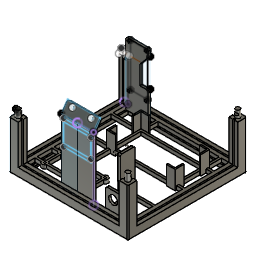
frame_base (Autodesk Fusion 360 design; units mm, degrees)
Autodesk Fusion 360 part; units mm, degrees
note: some values were not read from the file. Chosen so that the rebuilt part matches the saved one: which bodies a step acts on; a direction. Set by a fixed rule: which sketch regions a step uses; the direction of a hole.
sketch "Skizze1" plane through (0, 0, 0) normal (0, 0, 1) x (1, 0, 0)
  line L0 (0, 0) -> (160, 0)
  line L1 (160, 0) -> (160, 160)
  line L2 (160, 160) -> (0, 160)
  line L3 (0, 160) -> (0, 0)
  line L4 (12, 148) -> (148, 148)
  line L5 (148, 148) -> (148, 12)
  line L6 (148, 12) -> (12, 12)
  line L7 (12, 12) -> (12, 148)
  line L8 (12, 148) -> (0, 148)
  line L9 (0, 148) -> (0, 160)
  line L10 (0, 160) -> (12, 160)
  line L11 (12, 160) -> (12, 148)
  line L12 (148, 148) -> (160, 148)
  line L13 (160, 148) -> (160, 160)
  line L14 (160, 160) -> (148, 160)
  line L15 (148, 160) -> (148, 148)
  line L16 (148, 12) -> (160, 12)
  line L17 (160, 12) -> (160, 0)
  line L18 (160, 0) -> (148, 0)
  line L19 (148, 0) -> (148, 12)
  line L20 (12, 12) -> (0, 12)
  line L21 (0, 12) -> (0, 0)
  line L22 (0, 0) -> (12, 0)
  line L23 (12, 0) -> (12, 12)
  circle A0 centre (6, 6) radius 3
  circle A1 centre (154, 6) radius 3
  circle A2 centre (154, 154) radius 3
  circle A3 centre (6, 154) radius 3
  line L24 (154, 148) -> (154, 12) construction
  line L25 (148, 154) -> (12, 154) construction
  line L26 (6, 148) -> (6, 12) construction
  line L27 (12, 6) -> (148, 6) construction
  line L28 (152.9, 150) -> (155.1, 150)
  line L29 (155.1, 150) -> (155.1, 10)
  line L30 (155.1, 10) -> (152.9, 10)
  line L31 (152.9, 10) -> (152.9, 150)
  line L32 (4.9, 150) -> (7.1, 150)
  line L33 (7.1, 150) -> (7.1, 10)
  line L34 (7.1, 10) -> (4.9, 10)
  line L35 (4.9, 10) -> (4.9, 150)
  line L36 (10, 152.9) -> (150, 152.9)
  line L37 (150, 152.9) -> (150, 155.1)
  line L38 (150, 155.1) -> (10, 155.1)
  line L39 (10, 155.1) -> (10, 152.9)
  line L40 (10, 4.9) -> (150, 4.9)
  line L41 (150, 4.9) -> (150, 7.1)
  line L42 (150, 7.1) -> (10, 7.1)
  line L43 (10, 7.1) -> (10, 4.9)
  dimension "d1" = 160
  dimension "d2" = 160
  dimension "d3" = 12
  dimension "d4" = 12
  dimension "d5" = 12
  dimension "d6" = 12
  dimension "d7" = 6
  dimension "d8" = 6
  dimension "d9" = 6
  dimension "d10" = 6
  dimension "d11" = 6
  dimension "d12" = 6
  dimension "d13" = 6
  dimension "d14" = 6
  dimension "d15" = 6
  dimension "d16" = 6
  dimension "d17" = 6
  dimension "d18" = 6
  dimension "d19" = 2.2
  dimension "d20" = 140
  dimension "d21" = 4.9
  dimension "d22" = 10
  dimension "d23" = 2.2
  dimension "d24" = 140
  dimension "d25" = 4.9
  dimension "d26" = 10
  dimension "d27" = 140
  dimension "d28" = 2.2
  dimension "d29" = 10
  dimension "d30" = 4.9
  dimension "d31" = 140
  dimension "d32" = 2.2
  dimension "d33" = 10
  dimension "d34" = 4.9
  constraint horizontal L0
  constraint vertical L1
  constraint horizontal L2
  constraint vertical L3
  constraint coincident L0.start L3.end
  constraint horizontal L4
  constraint vertical L5
  constraint horizontal L6
  constraint vertical L7
  constraint horizontal L8
  constraint vertical L9
  constraint horizontal L10
  constraint vertical L11
  constraint horizontal L12
  constraint vertical L13
  constraint horizontal L14
  constraint vertical L15
  constraint horizontal L16
  constraint vertical L17
  constraint horizontal L18
  constraint vertical L19
  constraint horizontal L20
  constraint vertical L21
  constraint horizontal L22
  constraint vertical L23
  constraint midpoint L12 L24.start
  constraint midpoint L16 L24.end
  constraint midpoint L15 L25.start
  constraint midpoint L11 L25.end
  constraint midpoint L8 L26.start
  constraint midpoint L20 L26.end
  constraint midpoint L23 L27.start
  constraint midpoint L19 L27.end
  constraint horizontal L28
  constraint vertical L29
  constraint horizontal L30
  constraint vertical L31
  constraint horizontal L32
  constraint vertical L33
  constraint horizontal L34
  constraint vertical L35
  constraint horizontal L36
  constraint vertical L37
  constraint horizontal L38
  constraint vertical L39
  constraint horizontal L40
  constraint vertical L41
  constraint horizontal L42
  constraint vertical L43
  measures "d1" distance of L0.start L0.end
  measures "d2" distance of L0.start L2.end
  measures "d3" distance of L3 L7
  measures "d4" distance of L1 L5
  measures "d5" distance of L0 L6
  measures "d6" distance of L2 L4
  measures "d7" diameter of A0
  measures "d8" diameter of A1
  measures "d9" diameter of A2
  measures "d10" diameter of A3
  measures "d11" distance of L3 A0.centre
  measures "d12" distance of L17 A1.centre
  measures "d13" distance of L13 A2.centre
  measures "d14" distance of L3 A3.centre
  measures "d15" distance of L12 A2.centre
  measures "d16" distance of L0 A1.centre
  measures "d17" distance of L22 A0.centre
  measures "d18" distance of L8 A3.centre
  measures "d19" distance of L28.start L28.end
  measures "d20" distance of L28.start L30.end
  measures "d21" distance of L1 L29
  measures "d22" distance of L2 L28
  measures "d23" distance of L32.start L32.end
  measures "d24" distance of L32.start L34.end
  measures "d25" distance of L3 L35
  measures "d26" distance of L2 L32
  measures "d27" distance of L36.start L36.end
  measures "d28" distance of L36.start L38.end
  measures "d29" distance of L3 L39
  measures "d30" distance of L2 L38
  measures "d31" distance of L40.start L40.end
  measures "d32" distance of L40.start L42.end
  measures "d33" distance of L21 L43
  measures "d34" distance of L0 L40
ref_plane "Arbeitsebene1" through (80, 80, 7.1) normal (0, 0, 1) x (1, 0, 0)
sketch "Skizze2" plane through (80, 80, 7.1) normal (0, 0, 1) x (1, 0, 0)
  line L0 (-56, -33) -> (2.2, -33)
  line L1 (2.2, -33) -> (2.2, -56)
  line L2 (2.2, -56) -> (-56, -56)
  line L3 (-56, -56) -> (-56, -33)
  line L4 (-68, -68) -> (-68, 68)
  line L5 (68, -68) -> (-68, -68)
  line L6 (-54.5, -34.5) -> (0.7, -34.5)
  line L7 (0.7, -34.5) -> (0.7, -54.5)
  line L8 (0.7, -54.5) -> (-54.5, -54.5)
  line L9 (-54.5, -54.5) -> (-54.5, -34.5)
  line L10 (-57.5, -31.5) -> (3.7, -31.5)
  line L11 (3.7, -31.5) -> (3.7, -57.5)
  line L12 (3.7, -57.5) -> (-57.5, -57.5)
  line L13 (-57.5, -57.5) -> (-57.5, -31.5)
  circle A0 centre (-56, -33) radius 4
  circle A1 centre (2.2, -33) radius 4
  circle A2 centre (2.2, -56) radius 4
  circle A3 centre (-56, -56) radius 4
  line L14 (-57.5, -31.5) -> (-68, -31.5)
  line L15 (-68, -31.5) -> (-68, -34.5)
  line L16 (-68, -34.5) -> (-57.5, -34.5)
  line L17 (-57.5, -34.5) -> (-57.5, -31.5)
  line L18 (-57.5, -57.5) -> (-68, -57.5)
  line L19 (-68, -57.5) -> (-68, -54.5)
  line L20 (-68, -54.5) -> (-57.5, -54.5)
  line L21 (-57.5, -54.5) -> (-57.5, -57.5)
  line L22 (0, -68) -> (0, -65) construction
  line L23 (0, -65) -> (21.75, -65)
  line L24 (21.75, -65) -> (21.75, -68)
  line L25 (21.75, -68) -> (0, -68)
  line L26 (0, -65) -> (-21.75, -65)
  line L27 (-21.75, -65) -> (-21.75, -68)
  line L28 (-21.75, -68) -> (0, -68)
  line L29 (3.7, -57.5) -> (0.7, -57.5)
  line L30 (0.7, -57.5) -> (0.7, -65)
  line L31 (0.7, -65) -> (3.7, -65)
  line L32 (3.7, -65) -> (3.7, -57.5)
  line L33 (38, -65) -> (58, -65)
  line L34 (58, -65) -> (58, -68)
  line L35 (58, -68) -> (38, -68)
  line L36 (38, -68) -> (38, -65)
  line L37 (68, 68) -> (68, -68)
  line L38 (68, 68) -> (-68, 68) construction
  line L39 (-30.5, 48) -> (58, 48)
  line L40 (58, 48) -> (58, 5.5)
  line L41 (58, 5.5) -> (-30.5, 5.5)
  line L42 (-30.5, 5.5) -> (-30.5, 48)
  line L43 (-68, 68) -> (-38, 68)
  line L44 (-38, 68) -> (-38, 65)
  line L45 (-38, 65) -> (-68, 65)
  line L46 (-68, 65) -> (-68, 68)
  line L47 (-27.5, 45) -> (55, 45)
  line L48 (55, 45) -> (55, 8.5)
  line L49 (55, 8.5) -> (-27.5, 8.5)
  line L50 (-27.5, 8.5) -> (-27.5, 45)
  line L51 (-30.5, 48) -> (-20.5, 48)
  line L52 (-20.5, 48) -> (-20.5, 50)
  line L53 (-20.5, 50) -> (-30.5, 50)
  line L54 (-30.5, 50) -> (-30.5, 48)
  line L55 (-30.5, 5.5) -> (-20.5, 5.5)
  line L56 (-20.5, 5.5) -> (-20.5, 3.5)
  line L57 (-20.5, 3.5) -> (-30.5, 3.5)
  line L58 (-30.5, 3.5) -> (-30.5, 5.5)
  line L59 (58, 5.5) -> (48, 5.5)
  line L60 (48, 5.5) -> (48, 3.5)
  line L61 (48, 3.5) -> (58, 3.5)
  line L62 (58, 3.5) -> (58, 5.5)
  line L63 (58, 48) -> (48, 48)
  line L64 (48, 48) -> (48, 50)
  line L65 (48, 50) -> (58, 50)
  line L66 (58, 50) -> (58, 48)
  line L67 (-30.5, 50) -> (-32.5, 50)
  line L68 (-32.5, 50) -> (-32.5, 38)
  line L69 (-32.5, 38) -> (-30.5, 38)
  line L70 (-30.5, 38) -> (-30.5, 50)
  line L71 (-30.5, 3.5) -> (-32.5, 3.5)
  line L72 (-32.5, 3.5) -> (-32.5, 15.5)
  line L73 (-32.5, 15.5) -> (-30.5, 15.5)
  line L74 (-30.5, 15.5) -> (-30.5, 3.5)
  line L75 (58, 3.5) -> (60, 3.5)
  line L76 (60, 3.5) -> (60, 15.5)
  line L77 (60, 15.5) -> (58, 15.5)
  line L78 (58, 15.5) -> (58, 3.5)
  line L79 (58, 50) -> (60, 50)
  line L80 (60, 50) -> (60, 38)
  line L81 (60, 38) -> (58, 38)
  line L82 (58, 38) -> (58, 50)
  line L83 (60, 48) -> (68, 48)
  line L84 (68, 48) -> (68, 45)
  line L85 (68, 45) -> (60, 45)
  line L86 (60, 45) -> (60, 48)
  line L87 (60, 8.5) -> (68, 8.5)
  line L88 (68, 8.5) -> (68, 5.5)
  line L89 (68, 5.5) -> (60, 5.5)
  line L90 (60, 5.5) -> (60, 8.5)
  line L91 (58, 50) -> (55, 50)
  line L92 (55, 50) -> (55, 68)
  line L93 (55, 68) -> (58, 68)
  line L94 (58, 68) -> (58, 50)
  line L95 (-27.5, 50) -> (-30.5, 50)
  line L96 (-30.5, 50) -> (-30.5, 68)
  line L97 (-30.5, 68) -> (-27.5, 68)
  line L98 (-27.5, 68) -> (-27.5, 50)
  line L99 (-32.5, 5.5) -> (-68, 5.5)
  line L100 (-68, 5.5) -> (-68, 8.5)
  line L101 (-68, 8.5) -> (-32.5, 8.5)
  line L102 (-32.5, 8.5) -> (-32.5, 5.5)
  line L103 (-32.5, 45) -> (-68, 45)
  line L104 (-68, 45) -> (-68, 48)
  line L105 (-68, 48) -> (-32.5, 48)
  line L106 (-32.5, 48) -> (-32.5, 45)
  line L107 (-30.5, 3.5) -> (-27.5, 3.5)
  line L108 (-27.5, 3.5) -> (-27.5, -31.5)
  line L109 (-27.5, -31.5) -> (-30.5, -31.5)
  line L110 (-30.5, -31.5) -> (-30.5, 3.5)
  line L111 (38, -31.5) -> (41, -31.5)
  line L112 (41, -31.5) -> (41, -51.5)
  line L113 (41, -51.5) -> (38, -51.5)
  line L114 (38, -51.5) -> (38, -31.5)
  line L115 (38, -51.5) -> (41, -51.5)
  line L116 (41, -51.5) -> (41, -65)
  line L117 (41, -65) -> (38, -65)
  line L118 (38, -65) -> (38, -51.5)
  line L119 (41, -31.5) -> (68, -31.5)
  line L120 (68, -31.5) -> (68, -34.5)
  line L121 (68, -34.5) -> (41, -34.5)
  line L122 (41, -34.5) -> (41, -31.5)
  dimension "d36" = 58.2
  dimension "d37" = 23
  dimension "d38" = 12
  dimension "d39" = 12
  dimension "d40" = 55.2
  dimension "d41" = 20
  dimension "d42" = 1.5
  dimension "d43" = 1.5
  dimension "d44" = 61.2
  dimension "d45" = 26
  dimension "d46" = 1.5
  dimension "d47" = 1.5
  dimension "d48" = 8
  dimension "d49" = 8
  dimension "d50" = 8
  dimension "d51" = 8
  dimension "d52" = 10.5
  dimension "d53" = 3
  dimension "d54" = 10.5
  dimension "d55" = 3
  dimension "d56" = 3
  dimension "d57" = 21.75
  dimension "d58" = 3
  dimension "d59" = 3
  dimension "d60" = 7.5
  dimension "d61" = 20
  dimension "d62" = 3
  dimension "d63" = 10
  dimension "d64" = 3
  dimension "d65" = 88.5
  dimension "d66" = 42.5
  dimension "d67" = 30
  dimension "d68" = 3
  dimension "d69" = 10
  dimension "d70" = 20
  dimension "d71" = 82.5
  dimension "d72" = 36.5
  dimension "d73" = 3
  dimension "d74" = 3
  dimension "d75" = 10
  dimension "d76" = 2
  dimension "d77" = 10
  dimension "d78" = 2
  dimension "d79" = 10
  dimension "d80" = 2
  dimension "d81" = 10
  dimension "d82" = 2
  dimension "d83" = 2
  dimension "d84" = 12
  dimension "d85" = 2
  dimension "d86" = 12
  dimension "d87" = 2
  dimension "d88" = 12
  dimension "d89" = 2
  dimension "d90" = 12
  dimension "d91" = 3
  dimension "d92" = 3
  dimension "d93" = 3
  dimension "d94" = 18
  dimension "d95" = 3
  dimension "d96" = 18
  dimension "d97" = 82.5
  dimension "d98" = 20
  dimension "d99" = 36.5
  dimension "d100" = 3
  dimension "d101" = 3
  dimension "d102" = 3
  dimension "d103" = 35
  dimension "d104" = 20
  dimension "d105" = 36.5
  dimension "d106" = 8
  dimension "d107" = 8
  dimension "d108" = 3
  dimension "d109" = 20
  dimension "d110" = 106
  dimension "d111" = 36.5
  dimension "d112" = 3
  dimension "d113" = 3
  constraint horizontal L0
  constraint vertical L1
  constraint horizontal L2
  constraint vertical L3
  constraint horizontal L6
  constraint vertical L7
  constraint horizontal L8
  constraint vertical L9
  constraint horizontal L10
  constraint vertical L11
  constraint horizontal L12
  constraint vertical L13
  constraint coincident L0.start L3.end
  constraint coincident L0.end L1.start
  constraint coincident L1.end L2.start
  constraint coincident L2.end L3.start
  constraint horizontal L14
  constraint vertical L15
  constraint horizontal L16
  constraint vertical L17
  constraint horizontal L18
  constraint vertical L19
  constraint horizontal L20
  constraint vertical L21
  constraint midpoint L5 L22.start
  constraint perpendicular L5 L22
  constraint perpendicular L22 L23
  constraint perpendicular L23 L24
  constraint symmetric L25.end L22 L28.end
  constraint symmetric L23.start L22 L26.start
  constraint symmetric L22 L23.end L26.end
  constraint symmetric L22 L24.end L27.end
  constraint horizontal L29
  constraint vertical L30
  constraint horizontal L31
  constraint vertical L32
  constraint horizontal L33
  constraint vertical L34
  constraint horizontal L35
  constraint vertical L36
  constraint coincident L37.start L38.start
  constraint coincident L4.end L38.end
  constraint horizontal L39
  constraint vertical L40
  constraint horizontal L41
  constraint vertical L42
  constraint horizontal L43
  constraint vertical L44
  constraint horizontal L45
  constraint vertical L46
  constraint horizontal L47
  constraint vertical L48
  constraint horizontal L49
  constraint vertical L50
  constraint horizontal L51
  constraint vertical L52
  constraint horizontal L53
  constraint vertical L54
  constraint horizontal L55
  constraint vertical L56
  constraint horizontal L57
  constraint vertical L58
  constraint horizontal L59
  constraint vertical L60
  constraint horizontal L61
  constraint vertical L62
  constraint horizontal L63
  constraint vertical L64
  constraint horizontal L65
  constraint vertical L66
  constraint horizontal L67
  constraint vertical L68
  constraint horizontal L69
  constraint vertical L70
  constraint horizontal L71
  constraint vertical L72
  constraint horizontal L73
  constraint vertical L74
  constraint horizontal L75
  constraint vertical L76
  constraint horizontal L77
  constraint vertical L78
  constraint horizontal L79
  constraint vertical L80
  constraint horizontal L81
  constraint vertical L82
  constraint horizontal L83
  constraint vertical L84
  constraint horizontal L85
  constraint vertical L86
  constraint coincident L80 L83.start
  constraint horizontal L87
  constraint vertical L88
  constraint horizontal L89
  constraint vertical L90
  constraint coincident L76 L87.start
  constraint horizontal L91
  constraint vertical L92
  constraint horizontal L93
  constraint vertical L94
  constraint horizontal L95
  constraint vertical L96
  constraint horizontal L97
  constraint vertical L98
  constraint coincident L53 L95.start
  constraint horizontal L99
  constraint vertical L100
  constraint horizontal L101
  constraint vertical L102
  constraint coincident L72 L99.start
  constraint horizontal L103
  constraint vertical L104
  constraint horizontal L105
  constraint vertical L106
  constraint coincident L4 L104.end
  constraint coincident L68 L103.start
  constraint horizontal L107
  constraint vertical L108
  constraint horizontal L109
  constraint vertical L110
  constraint horizontal L111
  constraint vertical L112
  constraint horizontal L113
  constraint vertical L114
  constraint horizontal L115
  constraint vertical L116
  constraint horizontal L117
  constraint vertical L118
  constraint horizontal L119
  constraint vertical L120
  constraint horizontal L121
  constraint vertical L122
  measures "d36" distance of L0.start L0.end
  measures "d37" distance of L0.start L2.end
  measures "d38" distance of L3 L4
  measures "d39" distance of L2 L5
  measures "d40" distance of L6.start L6.end
  measures "d41" distance of L6.start L8.end
  measures "d42" distance of L2 L8
  measures "d43" distance of L3 L9
  measures "d44" distance of L10.start L10.end
  measures "d45" distance of L10.start L12.end
  measures "d46" distance of L3 L13
  measures "d47" distance of L2 L12
  measures "d48" diameter of A0
  measures "d49" diameter of A1
  measures "d50" diameter of A2
  measures "d51" diameter of A3
  measures "d52" distance of L10.start L14.end
  measures "d53" distance of L10.start L16.end
  measures "d54" distance of L12.end L18.end
  measures "d55" distance of L12.end L20.end
  measures "d56" distance of L22.start L22.end
  measures "d57" distance of L22.end L23.end
  measures "d58" distance of L23.end L24.end
  measures "d59" distance of L11.end L29.end
  measures "d60" distance of L11.end L31.end
  measures "d61" distance of L33.start L33.end
  measures "d62" distance of L33.start L35.end
  measures "d63" distance of L34 L37
  measures "d64" distance of L5 L33
  measures "d65" distance of L39.start L39.end
  measures "d66" distance of L39.start L41.end
  measures "d67" distance of L4.end L43.end
  measures "d68" distance of L4.end L45.end
  measures "d69" distance of L37 L40
  measures "d70" distance of L38 L39
  measures "d71" distance of L47.start L47.end
  measures "d72" distance of L47.start L49.end
  measures "d73" distance of L39 L47
  measures "d74" distance of L42 L50
  measures "d75" distance of L39.start L51.end
  measures "d76" distance of L39.start L53.end
  measures "d77" distance of L41.end L55.end
  measures "d78" distance of L41.end L57.end
  measures "d79" distance of L40.end L59.end
  measures "d80" distance of L40.end L61.end
  measures "d81" distance of L39.end L63.end
  measures "d82" distance of L39.end L65.end
  measures "d83" distance of L53.end L67.end
  measures "d84" distance of L53.end L69.end
  measures "d85" distance of L57.end L71.end
  measures "d86" distance of L57.end L73.end
  measures "d87" distance of L61.end L75.end
  measures "d88" distance of L61.end L77.end
  measures "d89" distance of L65.end L79.end
  measures "d90" distance of L65.end L81.end
  measures "d91" distance of L83.start L85.end
  measures "d92" distance of L87.start L89.end
  measures "d93" distance of L65.end L91.end
  measures "d94" distance of L65.end L93.end
  measures "d95" distance of L95.start L53.end
  measures "d96" distance of L95.start L97.end
  measures "d97" distance of L92 L98
  measures "d98" distance of L38 L83
  measures "d99" distance of L85 L87
  measures "d100" distance of L99.start L101.end
  measures "d101" distance of L103.start L105.end
  measures "d102" distance of L57.end L107.end
  measures "d103" distance of L57.end L109.end
  measures "d104" distance of L38 L105
  measures "d105" distance of L101 L103
  measures "d106" distance of L80 L84
  measures "d107" distance of L88 L90
  measures "d108" distance of L111.start L111.end
  measures "d109" distance of L111.start L113.end
  measures "d110" distance of L4 L114
  measures "d111" distance of L5 L111
  measures "d112" distance of L113.end L112.end
  measures "d113" distance of L111.end L121.end
extrude "Extrusion1" add sketch "Skizze1" along normal blind 12 contours L0 L19 L23 L40 | L3 L8 L20 L35 | L6 L19 L23 L42 | L7 L8 L20 L33 | L1 L12 L16 L29 | L2 L11 L15 L38 | L5 L12 L16 L31 | L4 L11 L15 L36 makes body 4 at (7.1, 102.6667, 8) makes body 4 at (57.3333, 152.9, 8) makes body 4 at (102.6667, 7.1, 8) makes body 4 at (148, 102.6667, 8) makes body 1 at (0, 102.6667, 8) makes body 3 at (102.6667, 160, 8) makes body 5 at (155.1, 102.6667, 8) makes body 2 at (57.3333, 4.9, 4)
extrude "Extrusion2" add sketch "Skizze1" along normal blind 75 separate body contours A0 | A1 | A2 | A3 makes body 6 at (151.2356, 152.8347, 50) makes body 7 at (153.0445, 3.1562, 25) makes body 8 at (3.1809, 155.0261, 50) makes body 9 at (8.9963, 5.8505, 50)
extrude "Extrusion3" add sketch "Skizze1" along normal blind 10 separate body contours L23 L40 L42 L43 | L20 L33 L34 L35 | L19 L40 L41 L42 | L8 L32 L33 L35 | L16 L29 L30 L31 | L11 L36 L38 L39 | L12 L28 L29 L31 | L15 L36 L37 L38 makes body 10 at (5.6333, 150, 3.3333) makes body 11 at (154.3667, 10, 6.6667) makes body 12 at (153.6333, 148, 6.6667) makes body 13 at (6.3667, 12, 3.3333) makes body 14 at (12, 154.3667, 6.6667) makes body 15 at (148, 5.6333, 3.3333) makes body 16 at (150, 153.6333, 6.6667) makes body 17 at (10, 6.3667, 3.3333)
extrude "Extrusion4" add sketch "Skizze1" along normal blind 10 separate body contours L19 L23 L40 L42 | L8 L20 L33 L35 | L12 L16 L29 L31 | L11 L15 L36 L38 makes body 18 at (152.9, 57.3333, 6.6667) makes body 19 at (4.9, 57.3333, 6.6667) makes body 20 at (102.6667, 155.1, 6.6667) makes body 21 at (102.6667, 7.1, 6.6667)
extrude "Extrusion5" add sketch "Skizze1" along normal blind 65 separate body contours L0 L3 L20 L21 L22 L23 L33 L34 L35 L40 L42 L43 | L0 L1 L16 L17 L18 L19 L29 L30 L31 L40 L41 L42 | L2 L3 L8 L9 L10 L11 L32 L33 L35 L36 L38 L39 | L1 L2 L12 L13 L14 L15 L28 L29 L31 L36 L37 L38 makes body 22 at (8.9851, 5.7013, 21.6667) makes body 23 at (151.2356, 152.8347, 43.3333) makes body 24 at (153.0445, 3.1562, 21.6667) makes body 25 at (3.1809, 155.0261, 43.3333)
sketch "Skizze3" plane through (0, 148, 0) normal (0, -1, 0) x (1, 0, 0)
  line L0 (12, 0) -> (148, 0)
  line L1 (148, 0) -> (148, 12)
  line L2 (148, 12) -> (12, 12)
  line L3 (12, 12) -> (12, 0)
  line L4 (10, 7.1) -> (150, 7.1)
  line L5 (150, 7.1) -> (150, 4.9)
  line L6 (150, 4.9) -> (10, 4.9)
  line L7 (10, 4.9) -> (10, 7.1)
  line L8 (0, 0) -> (160, 0)
  dimension "d124" = 140
  dimension "d125" = 2.2
  dimension "d126" = 4.9
  dimension "d127" = 2
  constraint horizontal L4
  constraint vertical L5
  constraint horizontal L6
  constraint vertical L7
  measures "d124" distance of L4.start L4.end
  measures "d125" distance of L4.start L6.end
  measures "d126" distance of L6 L8
  measures "d127" distance of L3 L7
extrude "Extrusion6" cut sketch "Skizze3" against normal blind 2 contours L3 L4 L6 L7 | L1 L3 L4 L6 | L1 L4 L5 L6 bodies 4 23 25
sketch "Skizze4" plane through (148, 0, 0) normal (-1, 0, 0) x (0, -1, 0)
  line L0 (-148, 0) -> (-12, 0)
  line L1 (-12, 0) -> (-12, 12)
  line L2 (-12, 12) -> (-148, 12)
  line L3 (-148, 12) -> (-148, 7.1)
  line L4 (-148, 7.1) -> (-148, 4.9)
  line L5 (-148, 4.9) -> (-148, 0)
  line L6 (-150, 7.1) -> (-10, 7.1)
  line L7 (-10, 7.1) -> (-10, 4.9)
  line L8 (-10, 4.9) -> (-150, 4.9)
  line L9 (-150, 4.9) -> (-150, 7.1)
  line L10 (-160, 0) -> (-148, 0)
  line L11 (-152.9, 0) -> (-152.9, 10)
  dimension "d130" = 140
  dimension "d131" = 2.2
  dimension "d132" = 4.9
  dimension "d133" = 2.9
  constraint horizontal L6
  constraint vertical L7
  constraint horizontal L8
  constraint vertical L9
  measures "d130" distance of L6.start L6.end
  measures "d131" distance of L6.start L8.end
  measures "d132" distance of L8 L10
  measures "d133" distance of L9 L11
extrude "Extrusion7" cut sketch "Skizze4" against normal blind 2 contours L4 L6 L8 L9 | L1 L4 L6 L8 | L1 L6 L7 L8 bodies 4 24
sketch "Skizze5" plane through (12, 0, 0) normal (1, 0, 0) x (0, 1, 0)
  line L0 (12, 0) -> (148, 0)
  line L1 (148, 0) -> (148, 4.9)
  line L2 (148, 4.9) -> (148, 7.1)
  line L3 (148, 7.1) -> (148, 12)
  line L4 (148, 12) -> (12, 12)
  line L5 (12, 12) -> (12, 0)
  line L6 (10, 7.1) -> (150, 7.1)
  line L7 (150, 7.1) -> (150, 4.9)
  line L8 (150, 4.9) -> (10, 4.9)
  line L9 (10, 4.9) -> (10, 7.1)
  line L10 (12, 0) -> (148, 0)
  dimension "d136" = 140
  dimension "d137" = 2.2
  dimension "d138" = 4.9
  dimension "d139" = 2
  constraint horizontal L6
  constraint vertical L7
  constraint horizontal L8
  constraint vertical L9
  measures "d136" distance of L6.start L6.end
  measures "d137" distance of L6.start L8.end
  measures "d138" distance of L8 L10
  measures "d139" distance of L5 L9
extrude "Extrusion8" cut sketch "Skizze5" against normal blind 2 contours L5 L6 L8 L9 | L2 L5 L6 L8 | L2 L6 L7 L8 bodies 4 22
sketch "Skizze6" plane through (0, 12, 0) normal (0, 1, 0) x (-1, 0, 0)
  line L0 (-148, 0) -> (-12, 0)
  line L1 (-12, 0) -> (-12, 4.9)
  line L2 (-12, 4.9) -> (-12, 7.1)
  line L3 (-12, 7.1) -> (-12, 12)
  line L4 (-12, 12) -> (-148, 12)
  line L5 (-148, 12) -> (-148, 7.1)
  line L6 (-148, 7.1) -> (-148, 4.9)
  line L7 (-148, 4.9) -> (-148, 0)
  line L8 (-150, 7.1) -> (-10, 7.1)
  line L9 (-10, 7.1) -> (-10, 4.9)
  line L10 (-10, 4.9) -> (-150, 4.9)
  line L11 (-150, 4.9) -> (-150, 7.1)
  line L12 (-148, 0) -> (-12, 0)
  dimension "d142" = 140
  dimension "d143" = 2.2
  dimension "d144" = 4.9
  dimension "d145" = 2
  constraint horizontal L8
  constraint vertical L9
  constraint horizontal L10
  constraint vertical L11
  measures "d142" distance of L8.start L8.end
  measures "d143" distance of L8.start L10.end
  measures "d144" distance of L10 L12
  measures "d145" distance of L7 L11
extrude "Extrusion9" cut sketch "Skizze6" against normal blind 2 contours L6 L8 L10 L11 | L2 L6 L8 L10 | L2 L8 L9 L10 bodies 4
extrude "Extrusion10" add sketch "Skizze2" along normal blind 4.9 separate body contours L10 L57 L107 L108 L109 L110 | L39 L40 L41 L42 L51 L55 L59 L63 L70 L74 L78 L82 | L4 L72 L99 L100 L101 L102 | L4 L68 L103 L104 L105 L106 | L53 L95 L96 L97 L98 | L37 L76 L87 L88 L89 L90 | L65 L91 L92 L93 L94 | L37 L80 L83 L84 L85 L86 | L33 L113 L115 L116 L117 L118 | L37 L112 L119 L120 L121 L122 makes body 26 at (142.6667, 128, 8.7333) makes body 27 at (23.8333, 88.5, 8.7333) makes body 28 at (135, 136, 8.7333) makes body 29 at (49.5, 60.1667, 8.7333) makes body 30 at (139, 45.5, 8.7333) makes body 31 at (142.6667, 88.5, 8.7333) makes body 32 at (23.8333, 128, 8.7333) makes body 33 at (49.5, 136, 8.7333) makes body 34 at (80, 86.5, 7.1) makes body 35 at (118, 19.5, 8.7333)
extrude "Extrusion11" add sketch "Skizze2" along normal blind 25 separate body contours L41 L55 L56 L57 L58 L74 L107 | L42 L58 L71 L72 L73 L74 L102 | L41 L59 L60 L61 L62 L78 | L42 L54 L67 L68 L69 L70 L106 | L40 L62 L75 L76 L77 L78 L90 | L39 L51 L52 L53 L54 L70 L95 | L40 L66 L79 L80 L81 L82 L86 | L39 L63 L64 L65 L66 L82 L91 makes body 36 at (55.5, 83.5, 15.4333) makes body 37 at (55.5, 130, 15.4333) makes body 38 at (132, 83.5, 15.4333) makes body 39 at (140, 126, 15.4333)
extrude "Extrusion12" add sketch "Skizze2" along normal blind 4.9 contours L0 L3 L10 L13 A0 L17 | L0 L3 L6 L9 A0 | L0 L10 A0 A1 L109 | L0 L6 A0 A1 | L3 L9 A0 A3 | L3 L13 A0 A3 | L0 L1 L10 L11 A1 | L0 L1 L6 L7 A1 | L10 A0 L14 | L6 L9 A0 | L2 L3 L8 L9 A3 | L2 L3 L12 L13 A3 L21 | L13 A0 L16 | L10 L11 A1 | L6 L7 A1 | L13 A0 L14 L16 L17 | L4 A0 L14 L15 L16 | L8 L9 A3 | L13 A3 L20 | L1 L11 A1 A2 | L1 L7 A1 A2 | L2 L8 A2 A3 | L2 L12 A2 A3 | L13 A3 L18 L20 L21 | L4 A3 L18 L19 L20 | L1 L2 L11 L12 A2 L29 | L1 L2 L7 L8 A2 | L7 L8 A2 | L12 A3 L18 | L11 A2 L32 | L12 A2 L30 | L12 A2 L29 L30 L32 | A2 L23 L30 L31 L32 bodies 29 10 11 12 13 14 15 16 17 18 19 20 21 22 23 24 25 26 27 28 30 31 32 33 36 37 38 39 4
extrude "Extrusion13" add sketch "Skizze2" along normal blind 85 separate body contours L5 L23 L24 L25 L26 L27 L28 L31 makes body 40
sketch "Skizze7" plane through (0, 12, 0) normal (0, -1, 0) x (1, 0, 0)
  line L0 (58.25, 7.1) -> (80, 7.1)
  line L1 (80, 7.1) -> (80, 92.1)
  line L2 (80, 92.1) -> (58.25, 92.1)
  line L3 (58.25, 92.1) -> (58.25, 7.1)
  line L4 (80, 92.1) -> (101.75, 92.1)
  line L5 (101.75, 7.1) -> (101.75, 92.1)
  line L6 (61.35, 88.5) -> (98.35, 88.5)
  line L7 (98.35, 88.5) -> (98.35, 55)
  line L8 (98.35, 55) -> (61.35, 55)
  line L9 (61.35, 55) -> (61.35, 88.5)
  line L10 (61.35, 84.25) -> (98.35, 84.25)
  line L11 (98.35, 84.25) -> (98.35, 59.25)
  line L12 (98.35, 59.25) -> (61.35, 59.25)
  line L13 (61.35, 59.25) -> (61.35, 84.25)
  circle A0 centre (61.35, 88.5) radius 1.6
  circle A1 centre (98.35, 84.25) radius 1.6
  circle A2 centre (98.35, 59.25) radius 1.6
  circle A3 centre (61.35, 55) radius 1.6
  line L14 (58.25, 92.1) -> (101.75, 92.1)
  line L15 (101.75, 92.1, 0) -> (101.75, 104.3873, -8.6036)
  line L16 (101.75, 104.3873, -8.6036) -> (58.25, 104.3873, -8.6036)
  line L17 (58.25, 104.3873, -8.6036) -> (58.25, 92.1, 0)
  circle A4 through (68.675, 100.7011, -6.0226) (66.6125, 101.6765, -6.7056) (66.6125, 99.7257, -5.3395)
  circle A5 through (94.075, 100.7011, -6.0226) (92.0125, 101.6765, -6.7056) (92.0125, 99.7257, -5.3395)
  dimension "d156" = 37
  dimension "d157" = 33.5
  dimension "d160" = 25
  dimension "d161" = 4.25
  dimension "d162" = 3.2
  dimension "d163" = 3.2
  dimension "d164" = 3.2
  dimension "d165" = 3.2
  dimension "d166" = 3.4
  dimension "d169" = 15
  dimension "d170" = 2.75
  dimension "d171" = 4.5
  dimension "d172" = 9.05
  dimension "d173" = 2.75
  dimension "d174" = 25.4
  dimension "d175" = 9.05
  dimension "d176" = 4.5
  constraint horizontal L6
  constraint vertical L7
  constraint horizontal L8
  constraint vertical L9
  constraint horizontal L10
  constraint vertical L11
  constraint horizontal L12
  constraint vertical L13
  constraint coincident L9 L10.start
  constraint coincident L6.start L9.end
  constraint coincident L10.end L11.start
  constraint coincident L11.end L12.start
  constraint coincident L8.end L9.start
  constraint coincident L2.end L3.start
  measures "d156" distance of L6.start L6.end
  measures "d157" distance of L6.start L8.end
  measures "d160" distance of L10.start L12.end
  measures "d161" distance of L6 L10
  measures "d162" diameter of A0
  measures "d163" diameter of A1
  measures "d164" diameter of A2
  measures "d165" diameter of A3
  measures "d166" distance of L5 L10.end
sketch "Skizze7 (curves on the plane with normal 0, -0.8192, 0.5736 at 52.8264 mm)" plane through (0, -31.2728, 30.3) normal (0, -0.819152, 0.573576) x (-1, 0, 0)
  line L0 (-80, -75.4439) -> (-58.25, -75.4439)
  line L1 (-80, -75.4439) -> (-101.75, -75.4439)
  line L2 (-58.25, -75.4439) -> (-101.75, -75.4439)
  line L3 (-101.75, -75.4439) -> (-101.75, -90.4439)
  line L4 (-101.75, -90.4439) -> (-58.25, -90.4439)
  line L5 (-58.25, -90.4439) -> (-58.25, -75.4439)
  circle A0 centre (-67.3, -85.9439) radius 1.375
  circle A1 centre (-92.7, -85.9439) radius 1.375
extrude "Extrusion15" add sketch "Skizze7 (curves on the plane with normal 0, -0.8192, 0.5736 at 52.8264 mm)" against normal blind 3 separate body makes body 41
extrude "Extrusion14" cut sketch "Skizze7" against normal blind 3 contours L8 L9 A3 | L8 L9 A3 | L7 L11 L12 A2 | L7 L12 A2 | L7 L11 A2 | L6 L9 A0 | L6 L9 A0 | L7 L10 A1 | L7 L10 L11 A1 | L7 L11 A1 bodies 40
extrude "Extrusion16" add sketch "Skizze2" along normal blind 30 separate body contours L5 L33 L34 L35 L36 L117 makes body 42
sketch "Skizze8" plane through (0, 12, 0) normal (0, -1, 0) x (1, 0, 0)
  line L0 (118, 7.1) -> (138, 7.1)
  line L1 (138, 7.1) -> (138, 37.1)
  line L2 (138, 37.1) -> (118, 37.1)
  line L3 (118, 37.1) -> (118, 7.1)
  circle A0 centre (128, 26.1) radius 6
  dimension "d181" = 12
  dimension "d182" = 10
  dimension "d183" = 11
  measures "d181" diameter of A0
  measures "d182" distance of L3 A0.centre
  measures "d183" distance of L2 A0.centre
extrude "Extrusion17" cut sketch "Skizze8" against normal blind 3 contours A0 bodies 42
extrude "Extrusion18" add sketch "Skizze2" along normal blind 60 contours L111 L112 L113 L114 L115 L122 bodies 30 42 35
sketch "Skizze9" plane through (118, 0, 0) normal (-1, 0, 0) x (0, -1, 0)
  line L0 (-48.5, 7.1) -> (-15, 7.1)
  line L1 (-15, 7.1) -> (-15, 12)
  line L2 (-15, 12) -> (-28.5, 12)
  line L3 (-28.5, 12) -> (-28.5, 67.1)
  line L4 (-28.5, 67.1) -> (-48.5, 67.1)
  line L5 (-48.5, 67.1) -> (-48.5, 7.1)
  line L6 (-47.5, 65.6) -> (-29.5, 65.6)
  line L7 (-29.5, 65.6) -> (-29.5, 63.6)
  line L8 (-29.5, 63.6) -> (-47.5, 63.6)
  line L9 (-47.5, 63.6) -> (-47.5, 65.6)
  line L10 (-47.5, 65.6) -> (-45.5, 65.6)
  line L11 (-45.5, 65.6) -> (-45.5, 33.6)
  line L12 (-45.5, 33.6) -> (-47.5, 33.6)
  line L13 (-47.5, 33.6) -> (-47.5, 65.6)
  line L14 (-29.5, 65.6) -> (-31.5, 65.6)
  line L15 (-31.5, 65.6) -> (-31.5, 33.6)
  line L16 (-31.5, 33.6) -> (-29.5, 33.6)
  line L17 (-29.5, 33.6) -> (-29.5, 65.6)
  circle A0 centre (-30.5, 64.6) radius 0.95
  circle A1 centre (-46.5, 64.6) radius 0.95
  dimension "d188" = 18
  dimension "d189" = 2
  dimension "d190" = 1.5
  dimension "d191" = 1
  dimension "d192" = 2
  dimension "d193" = 32
  dimension "d194" = 2
  dimension "d195" = 32
  dimension "d196" = 1.9
  dimension "d197" = 1.9
  dimension "d198" = 1
  dimension "d199" = 1
  dimension "d200" = 1
  dimension "d201" = 1
  constraint horizontal L6
  constraint vertical L7
  constraint horizontal L8
  constraint vertical L9
  constraint horizontal L10
  constraint vertical L11
  constraint horizontal L12
  constraint vertical L13
  constraint horizontal L14
  constraint vertical L15
  constraint horizontal L16
  constraint vertical L17
  measures "d188" distance of L6.start L6.end
  measures "d189" distance of L6.start L8.end
  measures "d190" distance of L4 L6
  measures "d191" distance of L3 L7
  measures "d192" distance of L6.start L10.end
  measures "d193" distance of L6.start L12.end
  measures "d194" distance of L6.end L14.end
  measures "d195" distance of L6.end L16.end
  measures "d196" diameter of A0
  measures "d197" diameter of A1
  measures "d198" distance of L9 A1.centre
  measures "d199" distance of L8 A1.centre
  measures "d200" distance of L6 A0.centre
  measures "d201" distance of L17 A0.centre
extrude "Extrusion19" add sketch "Skizze9" along normal blind 2 contours L6 L8 L9 L10 L11 L13 | L6 L8 L11 L15 | L8 L11 L12 L13 | L6 L7 L8 L14 L15 L17 | L8 L15 L16 L17 bodies 30
extrude "Extrusion20" add 2 faces at (118, 30.5705, 64.9087) (118, 46.3417, 64.4435) along direction (-1, 0, 0) blind 7 on bodies 30 bodies 30
extrude "Extrusion21" add sketch "Skizze2" along normal blind 85 separate body contours L4 L43 L44 L45 L46 makes body 43
sketch "Skizze10" plane through (0, 148, 0) normal (0, 1, 0) x (-1, 0, 0)
  line L0 (-42, 7.1) -> (-12, 7.1)
  line L1 (-12, 7.1) -> (-12, 92.1)
  line L2 (-12, 92.1) -> (-42, 92.1)
  line L3 (-42, 92.1) -> (-42, 7.1)
  line L4 (-38.5, 88.5) -> (-15.5, 88.5)
  line L5 (-15.5, 88.5) -> (-15.5, 30.5)
  line L6 (-15.5, 30.5) -> (-38.5, 30.5)
  line L7 (-38.5, 30.5) -> (-38.5, 88.5)
  line L8 (-27.5, 69.5) -> (-10.387, 69.5) construction
  circle A0 centre (-38.5, 88.5) radius 1.6
  circle A1 centre (-15.5, 88.5) radius 1.6
  circle A2 centre (-38.5, 30.5) radius 1.6
  circle A3 centre (-15.5, 30.5) radius 1.6
  line L9 (-27.5, 69.5) -> (-4.942, 69.5) construction
  line L10 (-42, 44.5) -> (-31, 44.5)
  line L11 (-31, 44.5) -> (-31, 69.5)
  line L12 (-31, 69.5) -> (-42, 82.6093)
  line L13 (-31, 69.5) -> (-13.887, 69.5) construction
  line L14 (-12, 12) -> (-7.1, 12)
  line L15 (-12, 12) -> (-9, 12)
  line L16 (-9, 12) -> (-9, 65)
  line L17 (-9, 65) -> (-12, 65)
  line L18 (-12, 65) -> (-12, 12)
  dimension "d208" = 23
  dimension "d209" = 58
  dimension "d210" = 3.5
  dimension "d211" = 3.6
  dimension "d216" = 3.2
  dimension "d217" = 3.2
  dimension "d218" = 3.2
  dimension "d219" = 3.2
  dimension "d221" = 14
  dimension "d222" = 11
  dimension "d223" = 25
  dimension "d224" = 130
  constraint horizontal L4
  constraint vertical L5
  constraint horizontal L6
  constraint vertical L7
  constraint horizontal L8
  constraint coincident L4.start L7.end
  constraint coincident L4.end L5.start
  constraint coincident L6.end L7.start
  constraint coincident L5.end L6.start
  constraint horizontal L9
  constraint coincident L3 L10.start
  constraint perpendicular L7 L10
  constraint perpendicular L10 L11
  constraint horizontal L13
  constraint coincident L3 L12.end
  constraint horizontal L15
  constraint vertical L16
  constraint horizontal L17
  constraint vertical L18
  constraint coincident L14.start L15.start
  measures "d208" distance of L4.start L4.end
  measures "d209" distance of L4.start L6.end
  measures "d210" distance of L3 L7
  measures "d211" distance of L2 L4
  measures "d216" diameter of A0
  measures "d217" diameter of A1
  measures "d218" diameter of A2
  measures "d219" diameter of A3
  measures "d221" distance of L6 L10
  measures "d222" distance of L3 L11
  measures "d223" distance of L10 L11.end
  measures "d224" angle of L12 L13
extrude "Extrusion23" add sketch "Skizze10" against normal blind 3 separate body contours L1 L14 L15 L16 L17 L18 makes body 44
extrude "Extrusion22" cut sketch "Skizze10" against normal blind 3 contours L3 L7 L10 L12 | L7 L10 L11 L12 | L6 L7 A2 | L6 L7 A2 | L4 L7 A0 | L4 L7 A0 | L5 L6 A3 | L5 L6 A3 | L4 L5 A1 | L4 L5 A1 bodies 43
sketch "Skizze11" plane through (0, 0, 0) normal (-1, 0, 0) x (0, -1, 0)
  line L0 (-12, 0) -> (0, 0)
  line L1 (0, 0) -> (0, 65)
  line L2 (0, 65) -> (-12, 65)
  line L3 (-12, 65) -> (-12, 0)
  line L4 (-12, 65) -> (-9, 65) construction
  line L5 (-9, 65) -> (-9, 70) construction
  circle A0 centre (-9, 70) radius 1.5
  line L6 (-148, 65) -> (-151, 65) construction
  line L7 (-151, 65) -> (-151, 70) construction
  circle A1 centre (-151, 70) radius 1.5
  dimension "d229" = 3
  dimension "d230" = 5
  dimension "d231" = 3
  dimension "d233" = 3
  dimension "d234" = 5
  dimension "d235" = 3
  constraint coincident L2.end L3.start
  constraint perpendicular L3 L4
  constraint perpendicular L4 L5
  constraint coincident L5.end A0.centre
  constraint horizontal L6
  constraint perpendicular L6 L7
  constraint coincident L7.end A1.centre
  measures "d229" distance of L2.end L4.end
  measures "d230" distance of L4.end L5.end
  measures "d231" diameter of A0
  measures "d233" distance of L6.start L6.end
  measures "d234" distance of L6.end L7.end
  measures "d235" diameter of A1
extrude "Extrusion25" cut sketch "Skizze11" against normal through all contours A1 bodies 6 8
extrude "Extrusion24" cut sketch "Skizze11" against normal through all contours A0 bodies 7 9
hole "Bohrung1" at (24, 24, 7.1) direction (0, 0, -1) diameter 25 depth 4.9 tip angle 180 counterbore diameter 27.5 counterbore depth 1 bodies 29
hole "Bohrung2" at (24, 24, 7.1) direction (0, 0, 1) diameter 2.75 depth 4.9 tip angle 180 counterbore diameter 5.55 counterbore depth 2.5 bodies 29
hole "Bohrung3" at (82.2, 24, 7.1) direction (0, 0, 1) diameter 2.75 depth 4.9 tip angle 180 counterbore diameter 5.55 counterbore depth 2.5 bodies 29
hole "Bohrung4" at (24, 47, 7.1) direction (0, 0, 1) diameter 2.75 depth 4.9 tip angle 180 counterbore diameter 5.55 counterbore depth 2.5 bodies 29
hole "Bohrung5" at (82.2, 47, 7.1) direction (0, 0, 1) diameter 2.75 depth 4.9 tip angle 180 counterbore diameter 5.55 counterbore depth 2.5 bodies 29
combine "Kombinieren2" operation add target body 1 tool bodies 15 7 11 22 25 14 20 8 3 28 16 39 41 42 34 31 10 9 26 23 43 37 32 29 44 38 17 40 36 33 13 27 21 makes body 45 at (153.1875, 3.1121, 50)
combine "Kombinieren3" operation add target body 45 tool bodies 2 18 12 24 30 19 6 5 1
fillet "Abrundung1" radius 2 8 edges at (118, 13.5, 37.1) (138, 13.5, 37.1) (101.75, 21.8324, 103.5269) (58.25, 21.8324, 103.5269) (119.5, 48.5, 67.1) (119.5, 28.5, 67.1) (12, 146.5, 92.1) (42, 146.5, 92.1) on bodies 45
fillet "Abrundung2" radius 1.5 7 edges at (0, 160, 32.5) (0, 80, 0) (80, 0, 0) (160, 0, 32.5) (160, 80, 0) (160, 160, 32.5) (80, 160, 0) on bodies 45
fillet "Abrundung3" radius 1.5 2 edges at (0.4393, 0.4393, 0.4393) (0, 0, 33.25) on bodies 45
move_face "Flächen versetzen1" offset -0.1 8 faces at (151.2074, 7.096, 70) (3.2074, 7.096, 70) (3.2074, 152.9038, 69.9874) (151.2074, 152.9038, 69.9874) (154.6569, 151.7364, 71.3068) (6.6569, 151.7364, 71.3068) (5.3603, 8.3115, 71.3327) (153.3603, 8.3115, 71.3327) on bodies 45
